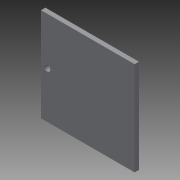
# Autodesk Inventor part: power_suply
Saved by Autodesk Inventor 2015 (Build 190159000, 159)
## iProperties
Created: 2015-07-30
Part Number: power_suply
Material: Generic
Document SubType Name: Modeling
Designer: Simen
Density: 1 g/cm^3
Appearance: Default
Author: Simen
Autodesk Inventor part; units mm, degrees
ref_plane "YZ Plane" through (0, 0, 0) normal (1, 0, 0) x (0, 1, 0)
ref_plane "XZ Plane" through (0, 0, 0) normal (0, 1, 0) x (-1, 0, 0)
ref_plane "XY Plane" through (0, 0, 0) normal (0, 0, 1) x (1, 0, 0)
sketch "Sketch1" plane through (0, 0, 0) normal (0, 1, 0) x (-1, 0, 0)
  line L0 (0, 0) -> (75, 0)
  line L1 (75, 0) -> (75, -75)
  line L2 (75, -75) -> (0, -75)
  line L3 (0, -75) -> (0, 0)
  dimension "d0" = 75
  dimension "d1" = 75
  constraints: 8 end point, 2 parallel, 1 horizontal, 1 perpendicular
  measures "d0" distance of L1.end L2.end
  measures "d1" distance of L0.end L1.end
extrude "Extrusion1" add sketch "Sketch1" along normal blind 3.5
sketch "Sketch2" plane through (0, 3.5, 0) normal (0, 1, 0) x (1, 0, 0)
  line L0 (-75, 0) -> (0, 0) projected
  line L1 (0, 0) -> (0, 75) projected
  line L2 (0, 75) -> (-75, 75) projected
  line L3 (-75, 75) -> (-75, 0) projected
  line L4 (-75, 75) -> (-75, 0) projected
  line L5 (0, 0) -> (0, 75) projected
  line L6 (-5, 5) -> (-75, 5)
  line L7 (-70, 75) -> (-70, 0)
  circle A0 centre (-70, 37.5) radius 2.5
  circle A1 centre (-5, 37.5) radius 2.5
  line L8 (-75, 37.5) -> (-7.5, 37.5)
  line L9 (-2.5, 37.5) -> (0, 37.5)
  line L10 (-5, 75) -> (-5, 40)
  line L11 (-5, 35) -> (-5, 5)
  dimension "d5" = 5
  dimension "d6" = 5
  dimension "d7" = 5
  constraints: 12 end point, 4 point on circle, 3 midpoint, 2 centre point, 1 parallel
  measures "d5" distance between parallel lines of L3 L7
  measures "d6" diameter of A0
  measures "d7" diameter of A1
extrude "Extrusion2" cut sketch "Sketch2" against normal blind 3.5 contours A0 L8 L7 | L7 L8 A0 | A0 L7 L8 | A1 | L7 A0 L8
sketch "Sketch3" plane through (0, 3.5, 0) normal (0, 1, 0) x (1, 0, 0)
  circle A0 centre (-70, 37.5) radius 2.5 projected
  circle A1 centre (-5, 37.5) radius 2.5 projected
  line L0 (-75, 0) -> (0, 0) projected
  line L1 (0, 0) -> (0, 75) projected
  line L2 (0, 75) -> (-75, 75) projected
  line L3 (-75, 75) -> (-75, 0) projected
  line L4 (-10, 10) -> (-10, 65)
  line L5 (-65, 65) -> (-65, 10)
  line L6 (-65, 65) -> (-65, 75)
  line L7 (0, 75) -> (-75, 75) projected
  line L8 (-65, 10) -> (-65, 0)
  line L9 (-75, 0) -> (0, 0) projected
  line L10 (-10, 10) -> (-10, 0)
  line L11 (-10, 65) -> (-10, 75)
  dimension "d10" = 10
  constraints: 12 end point, 6 point on line, 2 perpendicular
  measures "d10" distance between parallel lines of L3 L5
extrude "Extrusion3" add sketch "Sketch3" along normal blind 32 contours L8 L5 L6 L2 L11 L4 L10 L0
body "Solid1"
